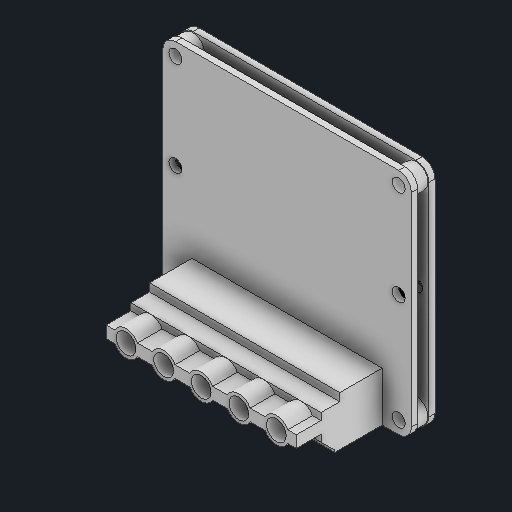
# Autodesk Inventor part: Driver
Saved by Autodesk Inventor 2025.1 (Build 291241020, 241B)
## iProperties
Created: 2025-09-06
Part Number: Driver
Material: 일반
Document SubType Name: Modeling
Designer: acalo
Density: 1 g/cm^3
Appearance: 기본값
Author: acalo
Autodesk Inventor part; units mm, degrees
ref_plane "YZ Plane" through (0, 0, 0) normal (1, 0, 0) x (0, 1, 0)
ref_plane "XZ Plane" through (0, 0, 0) normal (0, 1, 0) x (-1, 0, 0)
ref_plane "XY Plane" through (0, 0, 0) normal (0, 0, 1) x (1, 0, 0)
sketch "스케치8" plane through (0, 0, 0) normal (0, 0, 1) x (1, 0, 0)
  line L0 (-31.5, 29) -> (31.5, 29)
  line L1 (31.5, 29) -> (31.5, -29)
  line L2 (31.5, -29) -> (-31.5, -29)
  line L3 (-31.5, -29) -> (-31.5, 29)
  line L4 (-28.3, 25.75) -> (28.3, 25.75) construction
  line L5 (28.3, 25.75) -> (28.3, -25.75) construction
  line L6 (28.3, -25.75) -> (-28.3, -25.75) construction
  line L7 (-28.3, -25.75) -> (-28.3, 25.75) construction
  circle A0 centre (28.3, 25.75) radius 1.65
  circle A1 centre (-28.3, 25.75) radius 1.65
  circle A2 centre (-28.3, -25.75) radius 1.65
  circle A3 centre (28.3, -25.75) radius 1.65
  line L8 (-28.3, 25.75) -> (-28.3, 1.75) construction
  line L9 (-28.3, 1.75) -> (28.3, 1.75) construction
  circle A4 centre (-28.3, 1.75) radius 1.65
  circle A5 centre (28.3, 1.75) radius 1.65
  circle A6 centre (0, 0) radius 5
  dimension "d22" = 63
  dimension "d23" = 58
  dimension "d24" = 56.6
  dimension "d25" = 51.5
  dimension "d26" = 3.3
  dimension "d27" = 3.3
  dimension "d28" = 3.3
  dimension "d29" = 3.3
  dimension "d30" = 24
  dimension "d31" = 3.3
  dimension "d32" = 3.3
  dimension "d33" = 10
  constraints: 20 end point, 7 centre point, 4 parallel, 3 coincident, 3 perpendicular, 2 horizontal, 2 point on line
  measures "d22" distance of L1.end L2.end
  measures "d23" distance of L0.end L1.end
  measures "d24" distance of L5.end L6.end
  measures "d25" distance of L4.end L5.end
  measures "d26" diameter of A0
  measures "d27" diameter of A1
  measures "d28" diameter of A2
  measures "d29" diameter of A3
  measures "d30" distance of L8.start L8.end
  measures "d31" diameter of A4
  measures "d32" diameter of A5
  measures "d33" diameter of A6
extrude "돌출6" add sketch "스케치8" along normal blind 1.6
sketch "스케치9" plane through (0, 0, 1.6) normal (0, 0, 1) x (1, 0, 0)
  point P0 (0, 0)
fillet "모깎기1" radius 3.25 4 edges at (-31.5, -29, 0.8) (-31.5, 29, 0.8) (31.5, 29, 0.8) (31.5, -29, 0.8)
sketch "스케치10" plane through (0, 0, 1.6) normal (0, 0, 1) x (1, 0, 0)
  arc A0 (28.25, -29) -> (31.5, -25.75) centre (28.25, -25.75) ccw projected
  line L0 (31.5, -25.75) -> (31.5, 25.75) projected
  arc A1 (31.5, 25.75) -> (28.25, 29) centre (28.25, 25.75) ccw projected
  line L1 (28.25, 29) -> (-28.25, 29) projected
  arc A2 (-28.25, 29) -> (-31.5, 25.75) centre (-28.25, 25.75) ccw projected
  line L2 (-31.5, 25.75) -> (-31.5, -25.75) projected
  arc A3 (-31.5, -25.75) -> (-28.25, -29) centre (-28.25, -25.75) ccw projected
  line L3 (-28.25, -29) -> (28.25, -29) projected
  circle A4 centre (28.3, 25.75) radius 1.65 projected
  circle A5 centre (-28.3, 25.75) radius 1.65 projected
  circle A6 centre (-28.3, -25.75) radius 1.65 projected
  circle A7 centre (28.3, -25.75) radius 1.65 projected
  circle A8 centre (-28.3, 1.75) radius 1.65 projected
  circle A9 centre (28.3, 1.75) radius 1.65 projected
  circle A10 centre (0, 0) radius 5 construction
  circle A11 centre (28.3, -25.75) radius 3
  line L4 (0, 0) -> (0, -16) construction
  line L5 (0, 0) -> (-14, 0) construction
  circle A12 centre (-28.3, -25.75) radius 3
  circle A13 centre (28.3, 25.75) radius 3
  circle A14 centre (-28.3, 25.75) radius 3
  dimension "d37" = 6
  constraints: 4 centre point, 4 end point, 3 symmetric about line, 1 coincident, 1 horizontal, 1 vertical, 3 other
  measures "d37" diameter of A11
extrude "돌출7" add sketch "스케치10" along normal blind 2.8 contours A11 | A12 | A13 | A14
sketch "스케치11" plane through (28.3, 25.75, 4.4) normal (0, 0, 1) x (1, 0, 0)
  circle A0 centre (-56.6, -51.5) radius 3 projected
  circle A1 centre (-56.6, 0) radius 3 projected
  circle A2 centre (0, -51.5) radius 3 projected
  circle A3 centre (0, 0) radius 3 projected
  arc A4 (-0.05, -54.75) -> (3.2, -51.5) centre (-0.05, -51.5) ccw projected
  line L0 (3.2, -51.5) -> (3.2, 0) projected
  arc A5 (3.2, 0) -> (-0.05, 3.25) centre (-0.05, 0) ccw projected
  line L1 (-0.05, 3.25) -> (-56.55, 3.25) projected
  arc A6 (-56.55, 3.25) -> (-59.8, 0) centre (-56.55, 0) ccw projected
  line L2 (-59.8, 0) -> (-59.8, -51.5) projected
  arc A7 (-59.8, -51.5) -> (-56.55, -54.75) centre (-56.55, -51.5) ccw projected
  line L3 (-56.55, -54.75) -> (-0.05, -54.75) projected
  circle A8 centre (-56.6, -24) radius 1.65 projected
  circle A9 centre (0, -24) radius 1.65 projected
  circle A10 centre (-28.3, -25.75) radius 5 projected
  circle A11 centre (0, 0) radius 3 projected
  circle A12 centre (0, 0) radius 1.65 projected
  circle A13 centre (-56.6, 0) radius 3 projected
  circle A14 centre (-56.6, 0) radius 1.65 projected
  circle A15 centre (-56.6, -51.5) radius 1.65 projected
  circle A16 centre (0, -51.5) radius 1.65 projected
extrude "돌출8" add sketch "스케치11" along normal blind 1.6 contours A0 | A1 | A2 | A3 | L3 A7 L2 A6 L1 A5 L0 A4 | A10
sketch "스케치12" plane through (28.3, 25.75, 4.4) normal (0, 0, -1) x (-1, 0, 0)
  line L0 (25.6, -23.5) -> (31, -23.5)
  line L1 (31, -23.5) -> (31, -28)
  line L2 (31, -28) -> (25.6, -28)
  line L3 (25.6, -28) -> (25.6, -23.5)
  line L4 (25.6, -23.5) -> (31, -28) construction
  line L5 (31, -23.5) -> (25.6, -28) construction
  point P0 (28.3, -25.75)
  constraints: 12 end point, 2 midpoint, 2 parallel, 1 horizontal, 1 perpendicular
extrude "돌출9" add sketch "스케치12" along normal blind 1
sketch "스케치13" plane through (28.3, 25.75, 6) normal (0, 0, 1) x (1, 0, 0)
  line L0 (3.2, -51.5) -> (3.2, 0) projected
  arc A0 (3.2, 0) -> (-0.05, 3.25) centre (-0.05, 0) ccw projected
  line L1 (-0.05, 3.25) -> (-56.55, 3.25) projected
  arc A1 (-56.55, 3.25) -> (-59.8, 0) centre (-56.55, 0) ccw projected
  line L2 (-59.8, 0) -> (-59.8, -51.5) projected
  arc A2 (-59.8, -51.5) -> (-56.55, -54.75) centre (-56.55, -51.5) ccw projected
  line L3 (-56.55, -54.75) -> (-0.05, -54.75) projected
  arc A3 (-0.05, -54.75) -> (3.2, -51.5) centre (-0.05, -51.5) ccw projected
  circle A4 centre (-56.6, -51.5) radius 1.65 projected
  circle A5 centre (0, -51.5) radius 1.65 projected
  circle A6 centre (0, 0) radius 1.65 projected
  circle A7 centre (-56.6, 0) radius 1.65 projected
  circle A8 centre (-56.6, -24) radius 1.65 projected
  circle A9 centre (0, -24) radius 1.65 projected
  line L4 (-28.3, -54.75) -> (-28.3, -48.5)
  line L5 (-4.2, -42.25) -> (-52.4, -42.25)
  line L6 (-52.4, -42.25) -> (-52.4, -54.75)
  line L7 (-52.4, -54.75) -> (-4.2, -54.75)
  line L8 (-4.2, -54.75) -> (-4.2, -42.25)
  line L9 (-4.2, -42.25) -> (-52.4, -54.75) construction
  line L10 (-52.4, -42.25) -> (-4.2, -54.75) construction
  point P0 (-28.3, -25.75)
  dimension "d44" = 6.25
  dimension "d45" = 48.2
  constraints: 14 end point, 3 midpoint, 2 parallel, 1 horizontal, 1 perpendicular, 1 point on line, 1 vertical
  measures "d44" distance of L4.start L4.end
  measures "d45" distance of L7.end L6.end
extrude "돌출10" add sketch "스케치13" along normal blind 21.75 contours L3 L6 L5 L8
sketch "스케치14" plane through (28.3, 25.75, 27.75) normal (0, 0, 1) x (1, 0, 0)
  line L0 (-52.4, -42.25) -> (-52.4, -54.75) projected
  line L1 (-52.4, -54.75) -> (-4.2, -54.75) projected
  line L2 (-4.2, -54.75) -> (-4.2, -42.25) projected
  line L3 (-4.2, -42.25) -> (-52.4, -42.25) projected
  line L4 (-28.3, -42.25) -> (-28.3, -44.25)
  line L5 (-52.4, -44.25) -> (-4.2, -44.25)
  line L6 (-52.4, -50.75) -> (-4.2, -50.75)
  point P0 (-28.3, -25.75)
  constraints: 6 end point, 4 point on line, 2 midpoint, 1 perpendicular, 1 vertical
extrude "돌출11" cut sketch "스케치14" against normal blind 11 contours L3 L4 L5 L0 | L3 L2 L5 L4
extrude "돌출12" cut sketch "스케치14" against normal blind 9.75 contours L6 L2 L1 L0
chamfer "모따기1" distance 3.5 angle 45 1 edges at (0, -25, 18)
sketch "스케치15" plane through (28.3, 25.75, 27.75) normal (0, 0, 1) x (1, 0, 0)
  line L0 (-52.4, -50.75) -> (-4.2, -50.75) projected
  line L1 (-4.2, -50.75) -> (-4.2, -44.25) projected
  line L2 (-4.2, -44.25) -> (-52.4, -44.25) projected
  line L3 (-52.4, -44.25) -> (-52.4, -50.75) projected
  circle A0 centre (-28.3, -47.5) radius 3.25
  line L4 (-4.2, -47.5) -> (-6, -47.5)
  circle A1 centre (-9.25, -47.5) radius 3.25
  circle A2 centre (-18.775, -47.5) radius 3.25
  circle A3 centre (-47.35, -47.5) radius 3.25
  circle A4 centre (-37.825, -47.5) radius 3.25
  line L5 (-4.2, -46) -> (-52.4, -46)
  line L6 (-52.4, -49) -> (-4.2, -49)
  point P0 (-28.3, -25.75)
  point P1 (-6.3669, -49)
  point P2 (-9.25, -50.75)
  point P3 (-50.2331, -49)
  point P4 (-47.35, -50.75)
  point P5 (-40.7081, -49)
  point P6 (-44.4669, -49)
  point P7 (-37.825, -50.75)
  point P8 (-31.1831, -49)
  point P9 (-34.9419, -49)
  point P10 (-28.3, -50.75)
  point P11 (-21.6581, -49)
  point P12 (-25.4169, -49)
  point P13 (-18.775, -50.75)
  point P14 (-12.1331, -49)
  point P15 (-15.8919, -49)
  point P16 (-50.2331, -46)
  point P17 (-47.35, -44.25)
  point P18 (-44.4669, -46)
  point P19 (-40.7081, -46)
  point P20 (-37.825, -44.25)
  point P21 (-34.9419, -46)
  point P22 (-31.1831, -46)
  point P23 (-28.3, -44.25)
  point P24 (-25.4169, -46)
  point P25 (-21.6581, -46)
  point P26 (-18.775, -44.25)
  point P27 (-15.8919, -46)
  point P28 (-12.1331, -46)
  point P29 (-9.25, -44.25)
  point P30 (-6.3669, -46)
  dimension "d57" = 22.3
  constraints: 6 end point, 4 centre point, 4 point on line, 3 horizontal, 2 tangent, 1 midpoint, 1 parallel, 4 other
  measures "d57" distance of A0.centre L4.end
extrude "돌출13" cut sketch "스케치15" against normal blind 6.25 contours L3 L6 A3 L0 | A3 L6 A4 L0 | A4 L6 A0 L0 | L3 L2 A3 L5 | A0 L6 A2 L0 | A2 L6 A1 L0 | L5 A3 L2 A4 | A1 L6 L1 L0 | L5 A4 L2 A0 | L5 A0 L2 A2 | L5 A2 L2 A1 | L2 L1 L5 A1
sketch "스케치16" plane through (28.3, 25.75, 27.75) normal (0, 0, 1) x (1, 0, 0)
  arc A0 (-50.2331, -49) -> (-44.4669, -49) centre (-47.35, -47.5) ccw projected
  circle A1 centre (-47.35, -47.5) radius 2.5
  arc A2 (-40.7081, -49) -> (-34.9419, -49) centre (-37.825, -47.5) ccw projected
  line L0 (-47.35, -47.5) -> (-37.825, -47.5)
  circle A3 centre (-37.825, -47.5) radius 2.5
  circle A4 centre (-28.3, -47.5) radius 2.5
  circle A5 centre (-18.775, -47.5) radius 2.5
  circle A6 centre (-9.25, -47.5) radius 2.5
  point P0 (-28.3, -25.75)
  dimension "d60" = 5
  dimension "d63" = 9.525
  constraints: 5 centre point, 2 end point, 2 horizontal, 1 coincident, 8 other
  measures "d60" diameter of A1
  measures "d63" distance of L0.start A3.centre
extrude "돌출14" cut sketch "스케치16" against normal up to surface (6.25 mm away)
sketch "스케치17" plane through (-28.25, -29, 4.4) normal (0, -1, 0) x (1, 0, 0)
  line L0 (52.35, 13.6) -> (4.15, 13.6) projected
  line L1 (4.15, 1.6) -> (4.15, 13.6) projected
  line L2 (0, 1.6) -> (4.15, 1.6) projected
  line L3 (0, 0) -> (0, 1.6) projected
  line L4 (0, 0) -> (56.5, 0) projected
  line L5 (56.5, 0) -> (56.5, 1.6) projected
  line L6 (52.35, 1.6) -> (56.5, 1.6) projected
  line L7 (52.35, 1.6) -> (52.35, 13.6) projected
  line L8 (52.35, 1.6) -> (47.3, 1.6)
  line L9 (4.15, 1.6) -> (52.35, 1.6) projected
  line L10 (47.3, 6.5) -> (47.3, 1.6)
  line L11 (47.3, 6.5) -> (47.3, 9.1)
  line L12 (49.2, 11.7) -> (45.4, 11.7)
  line L13 (45.4, 11.7) -> (45.4, 6.5)
  line L14 (45.4, 6.5) -> (49.2, 6.5)
  line L15 (49.2, 6.5) -> (49.2, 11.7)
  line L16 (49.2, 11.7) -> (45.4, 6.5) construction
  line L17 (45.4, 11.7) -> (49.2, 6.5) construction
  line L18 (50.1831, 23.35) -> (44.4169, 23.35) projected
  line L19 (47.3, 23.35) -> (47.3, 27)
  line L20 (35.875, 11.7) -> (35.875, 6.5)
  line L21 (39.675, 11.7) -> (35.875, 11.7)
  line L22 (35.875, 11.7) -> (39.675, 6.5) construction
  line L23 (39.675, 11.7) -> (35.875, 6.5) construction
  line L24 (39.675, 6.5) -> (39.675, 11.7)
  line L25 (35.875, 6.5) -> (39.675, 6.5)
  line L26 (26.35, 11.7) -> (26.35, 6.5)
  line L27 (30.15, 11.7) -> (26.35, 11.7)
  line L28 (26.35, 11.7) -> (30.15, 6.5) construction
  line L29 (30.15, 11.7) -> (26.35, 6.5) construction
  line L30 (30.15, 6.5) -> (30.15, 11.7)
  line L31 (26.35, 6.5) -> (30.15, 6.5)
  line L32 (16.825, 11.7) -> (16.825, 6.5)
  line L33 (20.625, 11.7) -> (16.825, 11.7)
  line L34 (16.825, 11.7) -> (20.625, 6.5) construction
  line L35 (20.625, 11.7) -> (16.825, 6.5) construction
  line L36 (20.625, 6.5) -> (20.625, 11.7)
  line L37 (16.825, 6.5) -> (20.625, 6.5)
  line L38 (7.3, 11.7) -> (7.3, 6.5)
  line L39 (11.1, 11.7) -> (7.3, 11.7)
  line L40 (7.3, 11.7) -> (11.1, 6.5) construction
  line L41 (11.1, 11.7) -> (7.3, 6.5) construction
  line L42 (11.1, 6.5) -> (11.1, 11.7)
  line L43 (7.3, 6.5) -> (11.1, 6.5)
  point P0 (28.25, -4.4)
  point P1 (37.775, 9.1)
  point P2 (28.25, 9.1)
  point P3 (18.725, 9.1)
  point P4 (9.2, 9.1)
  dimension "d70" = 4.9
  dimension "d71" = 2.6
  dimension "d72" = 3.8
  dimension "d73" = 5.2
  dimension "d76" = 9.525
  constraints: 68 end point, 3 midpoint, 2 horizontal, 2 parallel, 2 perpendicular, 2 point on line, 2 vertical, 44 other
  measures "d70" distance of L10.start L8.end
  measures "d71" distance of L10.start L11.end
  measures "d72" distance of L14.end L13.end
  measures "d73" distance of L13.end L12.end
  measures "d76" distance of L12.end L20.start
extrude "돌출15" cut sketch "스케치17" against normal blind 8 contours L14 L13 L12 L15 | L21 L24 L25 L20 | L27 L30 L31 L26 | L33 L36 L37 L32 | L39 L42 L43 L38
sketch "스케치18" plane through (-28.25, -29, 4.4) normal (0, -1, 0) x (1, 0, 0)
  line L0 (11.1, 6.5) -> (7.3, 6.5) projected
  line L1 (11.1, 11.7) -> (11.1, 6.5) projected
  line L2 (7.3, 11.7) -> (11.1, 11.7) projected
  line L3 (7.3, 6.5) -> (7.3, 11.7) projected
  line L4 (12.1, 5.5) -> (6.3, 5.5)
  line L5 (6.3, 12.7) -> (12.1, 12.7)
  line L6 (5.1, 12.7) -> (13.3, 12.7)
  line L7 (13.3, 12.7) -> (13.3, 5.5)
  line L8 (13.3, 5.5) -> (5.1, 5.5)
  line L9 (5.1, 5.5) -> (5.1, 12.7)
  line L10 (13.3, 12.7) -> (5.1, 5.5) construction
  line L11 (21.625, 5.5) -> (15.825, 5.5)
  line L12 (15.825, 12.7) -> (21.625, 12.7)
  line L13 (14.625, 12.7) -> (22.825, 12.7)
  line L14 (22.825, 12.7) -> (22.825, 5.5)
  line L15 (22.825, 5.5) -> (14.625, 5.5)
  line L16 (14.625, 5.5) -> (14.625, 12.7)
  line L17 (31.15, 5.5) -> (25.35, 5.5)
  line L18 (25.35, 12.7) -> (31.15, 12.7)
  line L19 (24.15, 12.7) -> (32.35, 12.7)
  line L20 (32.35, 12.7) -> (32.35, 5.5)
  line L21 (32.35, 5.5) -> (24.15, 5.5)
  line L22 (24.15, 5.5) -> (24.15, 12.7)
  line L23 (40.675, 5.5) -> (34.875, 5.5)
  line L24 (34.875, 12.7) -> (40.675, 12.7)
  line L25 (33.675, 12.7) -> (41.875, 12.7)
  line L26 (41.875, 12.7) -> (41.875, 5.5)
  line L27 (41.875, 5.5) -> (33.675, 5.5)
  line L28 (33.675, 5.5) -> (33.675, 12.7)
  line L29 (50.2, 5.5) -> (44.4, 5.5)
  line L30 (44.4, 12.7) -> (50.2, 12.7)
  line L31 (43.2, 12.7) -> (51.4, 12.7)
  line L32 (51.4, 12.7) -> (51.4, 5.5)
  line L33 (51.4, 5.5) -> (43.2, 5.5)
  line L34 (43.2, 5.5) -> (43.2, 12.7)
  point P0 (28.25, -4.4)
  point P1 (9.2, 9.1)
  point P2 (50.2, 12.7)
  point P3 (44.4, 12.7)
  point P4 (31.15, 12.7)
  point P5 (25.35, 12.7)
  point P6 (12.1, 12.7)
  point P7 (6.3, 12.7)
  point P8 (6.3, 5.5)
  dimension "d84" = 8.2
  dimension "d87" = 9.525
  constraints: 62 end point, 2 horizontal, 2 parallel, 1 collinear, 1 midpoint, 1 perpendicular, 55 other
  measures "d84" distance of L7.end L8.end
  measures "d87" distance of L4.start L11.start
extrude "돌출16" cut sketch "스케치18" against normal blind 1.2
chamfer "모따기2" distance 1.2 distance2 2.2 1 edges at (-17.15, -27.8, 13.5) measured on face at (-17.15, -25.5333, 12.6333)
chamfer "모따기3" distance 1.2 distance2 2.2 1 edges at (-20.95, -27.8, 13.5) measured on face at (-20.95, -25.5333, 14.3667)
chamfer "모따기4" distance 1.2 distance2 1 1 edges at (-19.05, -27.8, 16.1) measured on face at (-19.6833, -24.7337, 16.1)
chamfer "모따기5" distance 1.2 distance2 1 1 edges at (-19.05, -27.8, 10.9) measured on face at (-19.6833, -24.7337, 10.9)
pattern_linear "직사각형 패턴1" count 5 spacing 9.525 along (1, 0, 0) of "모따기3", "모따기4", "모따기5", "돌출15", "모따기2", "돌출16"
